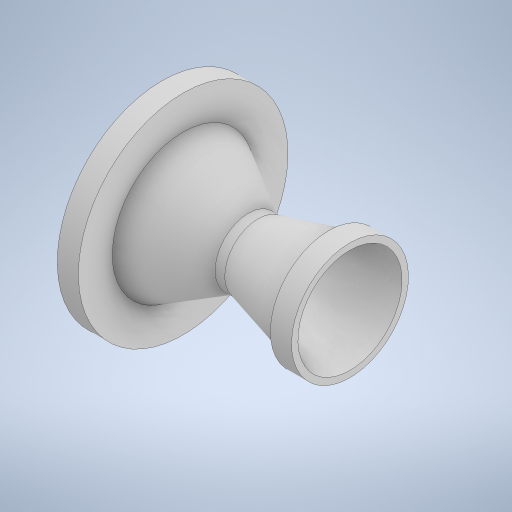
# Autodesk Inventor part: nozzle
Saved by Autodesk Inventor 2023 (Build 270158000, 158)
## iProperties
Created: 2022-09-14
Part Number: nozzle
Material: Generic
Document SubType Name: Modeling
Designer: station
Density: 1 g/cm^3
Appearance: Default
Author: station
Autodesk Inventor part; units mm, degrees
ref_plane "YZ Plane" through (0, 0, 0) normal (1, 0, 0) x (0, 1, 0)
ref_plane "XZ Plane" through (0, 0, 0) normal (0, 1, 0) x (-1, 0, 0)
ref_plane "XY Plane" through (0, 0, 0) normal (0, 0, 1) x (1, 0, 0)
sketch "Sketch1" plane through (0, 0, 0) normal (0, 0, 1) x (1, 0, 0)
  line L0 (0, 0) -> (0, 54.375)
  line L1 (0, 54.375) -> (192, 54.375)
  line L2 (0, 0) -> (772.3927, 0)
  line L3 (253.9225, 18.624) -> (253.9225, 0) construction
  line L4 (192, 54.375) -> (253.9225, 18.624)
  line L5 (253.9225, 18.624) -> (256.9225, 18.624)
  line L6 (256.9225, 18.624) -> (325.3908, 36.97)
  line L7 (325.3908, 36.97) -> (325.3908, 0)
  line L8 (192, 54.375) -> (192, 0)
  line L9 (0, 54.375) -> (0, 74.375)
  line L10 (0, 74.375) -> (20, 74.375)
  line L11 (20, 74.375) -> (20, 58.375)
  line L12 (192, 54.375) -> (192, 74.375)
  line L13 (192, 74.375) -> (172, 74.375)
  line L14 (172, 74.375) -> (172, 58.375)
  line L15 (20, 58.375) -> (172, 58.375)
  line L16 (192, 54.375) -> (192, 74.375)
  line L17 (192, 54.375) -> (192, 74.375)
  line L18 (192, 74.375) -> (207, 74.375)
  line L19 (325.3908, 36.4995) -> (325.3908, 41.4995)
  line L20 (207, 50.3335) -> (253.2623, 23.624)
  line L21 (260.128, 23.624) -> (310.3908, 37.0919)
  line L22 (253.2623, 23.624) -> (260.128, 23.624)
  line L23 (310.3908, 41.4995) -> (310.3908, 37.0919)
  line L24 (207, 74.375) -> (207, 50.3335)
  line L25 (207, 45.7147) -> (207, 21.1203)
  line L26 (325.3908, 36.4995) -> (325.3908, 41.4995)
  line L27 (325.3908, 41.4995) -> (310.3908, 41.4995)
  point P0 (255.4225, 18.624)
  dimension "d0" = 54.375
  dimension "d1" = 192
  dimension "d2" = 18.624
  dimension "d3" = 150
  dimension "d4" = 3
  dimension "d5" = 15
  dimension "d6" = 36.97
  dimension "d7" = 518.4701
  dimension "d8" = 20
  dimension "d9" = 20
  dimension "d10" = 16
  dimension "d11" = 20
  dimension "d12" = 20
  dimension "d13" = 16
  dimension "d14" = 20
  dimension "d15" = 15
  dimension "d18" = 4
  dimension "d21" = 5
  dimension "d22" = 15
  constraints: 56 end point, 13 perpendicular, 5 point on line, 3 horizontal, 3 vertical, 1 collinear, 1 midpoint, 1 parallel
  measures "d0" distance of L0.start L1.start
  measures "d1" distance of L1.start L8.start
  measures "d2" distance of L4.end L3.end
  measures "d3" angle of L4 L1
  measures "d4" distance of L4.end L5.end
  measures "d5" angle of L2 L6
  measures "d6" distance of L6.end L7.end
  measures "d7" distance from line of L2.end L3
  measures "d8" distance of L1.start L10.start
  measures "d9" distance of L10.start L11.start
  measures "d10" distance of L11.start L15.start
  measures "d11" distance of L8.start L12.end
  measures "d12" distance of L12.end L13.end
  measures "d13" distance of L13.end L14.end
  measures "d14" distance of L8.start L12.end
  measures "d15" distance of L12.end L18.end
  measures "d18" distance between parallel lines of L4 L20
  measures "d21" distance of L19.end L19.start
  measures "d22" distance of L19.end L23.start
revolve "Revolution1" add sketch "Sketch1" angle 360 about axis through (0, 0, 0) along (1, 0, 0) contours L12 L18 L24 L20 L22 L21 L23 L27 L19 L6 L5 L4
body "Solid1"
